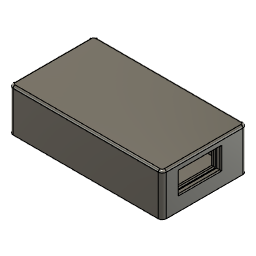
AC (Autodesk Fusion 360 design; units mm, degrees)
Autodesk Fusion 360 part; units mm, degrees
note: some values were not read from the file. Set by a fixed rule: which sketch regions a step uses.
sketch "Sketch1" plane through (0, 0, 0) normal (0, 1, 0) x (1, 0, 0) in component "Body"
  line L0 (0, 0) -> (72, 0)
  line L1 (72, 0) -> (72, 38)
  line L2 (72, 38) -> (0, 38)
  line L3 (0, 38) -> (0, 0)
  dimension "d1" = 72
  dimension "d2" = 38
  constraint horizontal L0
  constraint vertical L1
  constraint horizontal L2
  constraint vertical L3
  constraint coincident L0.start L3.end
  measures "d1" distance of L0.start L0.end
  measures "d2" distance of L0.start L2.end
extrude "Extrude1" add sketch "Sketch1" along normal blind 20 makes body 1 in component "Body"
shell "Shell2" thickness 1.6 removed faces 1 at (24, 20, -25.3333) on bodies 1 in component "Body"
sketch "Sketch2" plane through (0, 0, 0) normal (-1, 0, 0) x (0, 0, 1) in component "Body"
  line L0 (-38, 0) -> (0, 0)
  line L1 (0, 0) -> (0, 20)
  line L2 (0, 20) -> (-38, 20)
  line L3 (-38, 20) -> (-38, 0)
  circle A0 centre (-21.5264, 6.7451) radius 3.25
  line L4 (-4.7878, 9.0349) -> (-9.997, 9.0705)
  arc A1 (-9.997, 9.0705) -> (-4.7878, 9.0349) centre (-7.4057, 7.1089) ccw
  dimension "d12" = 6.5
  dimension "d13" = 6.5
  measures "d12" diameter of A1
  measures "d13" diameter of A0
extrude "Extrude4" cut sketch "Sketch2" against normal blind 2 contours A0 | L4 A1 bodies 1 in component "Body"
sketch "Sketch3" plane through (72, 0, 0) normal (1, 0, 0) x (0, 0, -1) in component "Body"
  line L0 (0, 0) -> (38, 0)
  line L1 (38, 0) -> (38, 20)
  line L2 (38, 20) -> (0, 20)
  line L3 (0, 20) -> (0, 0)
  line L4 (7.5322, 15.8374) -> (25.8872, 15.8374)
  line L5 (25.8872, 15.8374) -> (25.8872, 7.884)
  line L6 (25.8872, 7.884) -> (7.5322, 7.884)
  line L7 (7.5322, 7.884) -> (7.5322, 15.8374)
  constraint horizontal L4
  constraint vertical L5
  constraint horizontal L6
  constraint vertical L7
extrude "Extrude5" cut sketch "Sketch3" against normal blind 2 contours L4 L5 L6 L7 bodies 1 in component "Body"
fillet "Fillet1" radius 0.5 4 edges at (72, 11.8607, -7.5322) (72, 7.884, -16.7097) (72, 11.8607, -25.8872) (72, 15.8374, -16.7097) on bodies 1 in component "Body"
fillet "Fillet2" radius 0.6 4 edges at (72, 20, -19) (36, 20, -38) (0, 20, -19) (36, 20, 0) on bodies 1 in component "Body"
fillet "Fillet3" radius 0.2 4 edges at (36, 20, -1.6) (1.6, 20, -19) (36, 20, -36.4) (70.4, 20, -19) on bodies 1 in component "Body"
fillet "Fillet4" radius 0.2 4 edges at (70.4, 7.884, -16.7097) (70.4, 11.8607, -25.8872) (70.4, 15.8374, -16.7097) (70.4, 11.8607, -7.5322) on bodies 1 in component "Body"
fillet "Fillet5" radius 0.5 2 edges at (1.6, 3.859, -7.428) (1.6, 9.0527, -7.3924) on bodies 1 in component "Body"
fillet "Fillet6" radius 0.5 1 edges at (1.6, 5.5698, -24.5564) on bodies 1 in component "Body"
fillet "Fillet7" radius 0.2 3 edges at (0, 7.9203, -24.5564) (0, 9.0527, -7.3924) (0, 3.859, -7.428) on bodies 1 in component "Body"
sketch "Sketch1 (2)" plane through (0, 1.6, 0) normal (0, 1, 0) x (-1, 0, 0) in component "Lid"
  line L0 (-1.6, -36.4) -> (-1.6, -1.6)
  line L1 (-1.6, -1.6) -> (-70.4, -1.6)
  line L2 (-70.4, -1.6) -> (-70.4, -36.4)
  line L3 (-70.4, -36.4) -> (-1.6, -36.4)
  line L4 (0, 0) -> (-72, 0) construction
  line L5 (2, 2) -> (-74.0031, 2)
  line L6 (-74.0031, 2) -> (-74.0031, -40.0063)
  line L7 (-74.0031, -40.0063) -> (2, -40.0063)
  line L8 (2, -40.0063) -> (2, 2)
  point P0 (-72, -38)
  constraint horizontal L5
  constraint vertical L6
  constraint horizontal L7
  constraint vertical L8
extrude "Extrude1'" add sketch "Sketch1 (2)" along normal blind 19 and the other way blind 2 separate body contours L0 L1 L2 L3 | L5 L6 L7 L8 makes body 2 in component "Lid"
shell "Shell1" thickness 2 removed faces 1 at (48.6687, -0.4, -12.0021) on bodies 2 in component "Lid"
sketch "Sketch2 (2)" plane through (-2, 0, 0) normal (-1, 0, 0) x (0, 0, 1) in component "Lid"
  line L0 (2, -0.4) -> (2, 20.6)
  line L1 (2, 20.6) -> (-40.0063, 20.6)
  line L2 (-40.0063, 20.6) -> (-40.0063, -0.4)
  line L3 (-40.0063, -0.4) -> (2, -0.4)
  line L4 (-25.2468, 10.8764) -> (-17.7468, 10.8764)
  line L5 (-17.7468, 10.8764) -> (-17.7468, -0.5236)
  line L6 (-17.7468, -0.5236) -> (-25.2468, -0.5236)
  line L7 (-25.2468, -0.5236) -> (-25.2468, 10.8764)
  line L8 (-11.1427, 10.9194) -> (-3.6427, 10.9194)
  line L9 (-3.6427, 10.9194) -> (-3.6427, -0.4806)
  line L10 (-3.6427, -0.4806) -> (-11.1427, -0.4806)
  line L11 (-11.1427, -0.4806) -> (-11.1427, 10.9194)
  dimension "d33" = 7.5
  dimension "d34" = 11.4
  dimension "d35" = 7.5
  dimension "d36" = 11.4
  constraint horizontal L4
  constraint vertical L5
  constraint horizontal L6
  constraint vertical L7
  constraint horizontal L8
  constraint vertical L9
  constraint horizontal L10
  constraint vertical L11
  measures "d33" distance of L4.start L4.end
  measures "d34" distance of L4.start L6.end
  measures "d35" distance of L8.start L8.end
  measures "d36" distance of L8.start L10.end
extrude "Extrude2" cut sketch "Sketch2 (2)" against normal blind 2 contours L3 L9 L10 L11 | L3 L8 L9 L11 | L3 L5 L6 L7 | L3 L4 L5 L7 bodies 2 in component "Lid"
sketch "Sketch3 (2)" plane through (74.0031, 0, 0) normal (1, 0, 0) x (0, 0, -1) in component "Lid"
  line L0 (40.0063, -0.4) -> (40.0063, 20.6)
  line L1 (40.0063, 20.6) -> (-2, 20.6)
  line L2 (-2, 20.6) -> (-2, -0.4)
  line L3 (-2, -0.4) -> (40.0063, -0.4)
  line L4 (27, 6.905) -> (6.4235, 6.905)
  line L5 (6.4235, 6.905) -> (6.4235, 17)
  line L6 (6.4235, 17) -> (27, 17)
  line L7 (27, 17) -> (27, 6.905)
  constraint horizontal L4
  constraint vertical L5
  constraint horizontal L6
  constraint vertical L7
extrude "Extrude5'" cut sketch "Sketch3 (2)" against normal blind 2 contours L4 L5 L6 L7 bodies 2 in component "Lid"
fillet "Fillet1'" radius 0.5 6 edges at (-2, 10.8764, -21.4968) (-2, 5.2382, -25.2468) (-2, 5.2382, -17.7468) (-2, 5.2597, -11.1427) (-2, 10.9194, -7.3927) (-2, 5.2597, -3.6427) on bodies 2 in component "Lid"
fillet "Fillet2'" radius 0.5 4 edges at (74.0031, 11.9525, -27) (74.0031, 17, -16.7118) (74.0031, 11.9525, -6.4235) (74.0031, 6.905, -16.7118) on bodies 2 in component "Lid"
fillet "Fillet3'" radius 2 4 edges at (-2, 10.1, 2) (-2, 10.1, -40.0063) (74.0031, 10.1, -40.0063) (74.0031, 10.1, 2) on bodies 2 in component "Lid"
fillet "Fillet4'" radius 1 8 edges at (73.4173, 20.6, -39.4205) (36.0015, 20.6, -40.0063) (-1.4142, 20.6, -39.4205) (-2, 20.6, -19.0031) (-1.4142, 20.6, 1.4142) (36.0015, 20.6, 2) (73.4173, 20.6, 1.4142) (74.0031, 20.6, -19.0031) on bodies 2 in component "Lid"
component "Body" placed x (1, 0, 0) y (0, 1, 0) z (0, 0, 1) at (0, 0, 0)
component "Lid" placed x (1, 0, 0) y (0, 1, 0) z (0, 0, 1) at (0, 0, 0)
